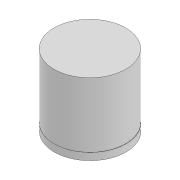
# Autodesk Inventor part: cyl1_10cm_10cm
Saved by Autodesk Inventor 2021 (Build 250183000, 183)
## iProperties
Created: 2023-09-29
Part Number: cyl1_10cm_10cm
Material: Generic
Document SubType Name: Modeling
Designer: eric5
Density: 1 g/cm^3
Appearance: Default
Author: eric5
Autodesk Inventor part; units mm, degrees
ref_plane "YZ Plane" through (0, 0, 0) normal (1, 0, 0) x (0, 1, 0)
ref_plane "XZ Plane" through (0, 0, 0) normal (0, 1, 0) x (-1, 0, 0)
ref_plane "XY Plane" through (0, 0, 0) normal (0, 0, 1) x (1, 0, 0)
sketch "Sketch2" plane through (0, 0, 0) normal (0, 1, 0) x (-1, 0, 0)
  point P0 (0, 0)
sketch "Sketch3" plane through (0, 0, 0) normal (0, 1, 0) x (-1, 0, 0)
  circle A0 centre (-0.2876, 0) radius 50
  point P0 (0, 0)
  dimension "d0" = 100
  constraints: 1 centre point
  measures "d0" diameter of A0
extrude "Extrusion1" add sketch "Sketch3" along normal blind 10
sketch "Sketch4" plane through (0.2876, 10, 0) normal (0, 1, 0) x (1, 0, 0)
  circle A0 centre (-0.2876, 0) radius 50.0008
  circle A1 centre (-0.2876, 0) radius 45
  circle A2 centre (-0.2876, 0) radius 10
  dimension "d3" = 90
  dimension "d4" = 20
  constraints: 3 centre point, 3 coincident
  measures "d3" diameter of A1
  measures "d4" diameter of A2
extrude "Extrusion2" add sketch "Sketch4" along normal blind 80
sketch "Sketch5" plane through (0, 90, 0) normal (0, 1, 0) x (1, 0, 0)
  circle A0 centre (0, 0) radius 50.0008
  constraints: 1 centre point, 1 coincident
extrude "Extrusion3" add sketch "Sketch5" along normal blind 10
body "Solid1"
